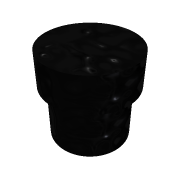
# Autodesk Inventor part: 00_Eyepiece_20x_WF
Saved by Autodesk Inventor 2019 (Build 230136000, 136)
## iProperties
Created: 2019-10-29
Part Number: 00_Eyepiece_20x_WF
Material: Generic
Document SubType Name: Modeling
Designer: diederichbenedict
Density: 1 g/cm^3
Appearance: Black
Author: diederichbenedict
Autodesk Inventor part; units mm, degrees
ref_plane "YZ Plane" through (0, 0, 0) normal (1, 0, 0) x (0, 1, 0)
ref_plane "XZ Plane" through (0, 0, 0) normal (0, 1, 0) x (-1, 0, 0)
ref_plane "XY Plane" through (0, 0, 0) normal (0, 0, 1) x (1, 0, 0)
sketch "Sketch1" plane through (0, 0, 0) normal (0, 0, 1) x (1, 0, 0)
  line L0 (0, 0) -> (11.5, 0)
  line L1 (11.5, 0) -> (11.5, 16.2)
  line L2 (11.5, 16.2) -> (13.9, 16.2)
  line L3 (13.9, 16.2) -> (13.9, 26.8)
  line L4 (13.9, 26.8) -> (0, 26.8)
  line L5 (0, 26.8) -> (0, 0)
  dimension "d0" = 11.5
  dimension "d1" = 16.2
  dimension "d2" = 2.4
  dimension "d3" = 10.6
  constraints: 12 end point, 5 perpendicular, 1 horizontal
  measures "d0" distance of L0.start L0.end
  measures "d1" distance of L0.end L1.end
  measures "d2" distance of L1.end L2.end
  measures "d3" distance of L2.end L3.end
revolve "Revolution1" add sketch "Sketch1" angle 360 about axis through (0, 26.8, 0) along (0, -1, 0)
body "Solid1"
